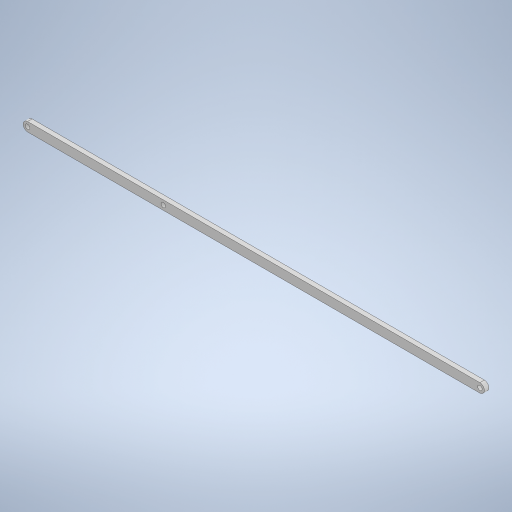
# Autodesk Inventor part: BCD
Saved by Autodesk Inventor 2024 (Build 280153000, 153)
## iProperties
Created: 2025-09-18
Part Number: BCD
Material: Generic
Document SubType Name: Modeling
Designer: Hello
Density: 1 g/cm^3
Appearance: Default
Author: Hello
Autodesk Inventor part; units mm, degrees
ref_plane "YZ Plane" through (0, 0, 0) normal (1, 0, 0) x (0, 1, 0)
ref_plane "XZ Plane" through (0, 0, 0) normal (0, 1, 0) x (-1, 0, 0)
ref_plane "XY Plane" through (0, 0, 0) normal (0, 0, 1) x (1, 0, 0)
sketch "Sketch1" plane through (0, 0, 0) normal (0, 0, 1) x (1, 0, 0)
  circle A0 centre (0, 0) radius 5
  arc A1 (0, 10) -> (0, -10) centre (0, 0) ccw
  line L0 (0, 0) -> (200, 0)
  circle A2 centre (1000, 0) radius 5
  arc A3 (1000, -10) -> (1000, 10) centre (1000, 0) ccw
  line L1 (0, 10) -> (1000, 10)
  line L2 (0, -10) -> (1000, -10)
  dimension "d0" = 10
  dimension "d1" = 20
  dimension "d3" = 10
  dimension "d4" = 20
  dimension "d7" = 1000
  constraints: 6 end point, 4 centre point, 4 point on circle, 3 coincident, 2 tangent, 1 horizontal
  measures "d0" diameter of A0
  measures "d1" diameter of A1
  measures "d3" diameter of A2
  measures "d4" diameter of A3
  measures "d7" distance of A2.centre A0.centre
extrude "Extrusion1" add sketch "Sketch1" along normal blind 10
sketch "Sketch2" plane through (0, 0, 10) normal (0, 0, 1) x (1, 0, 0)
  arc A0 (0, 10) -> (0, -10) centre (0, 0) ccw projected
  line L0 (0, 0) -> (300, 0)
  circle A1 centre (300, 0) radius 5
  dimension "d8" = 300
  dimension "d9" = 10
  constraints: 2 end point, 1 centre point, 1 coincident, 1 horizontal
  measures "d8" distance of L0.start L0.end
  measures "d9" diameter of A1
extrude "Extrusion2" cut sketch "Sketch2" against normal blind 10
body "Solid1"
